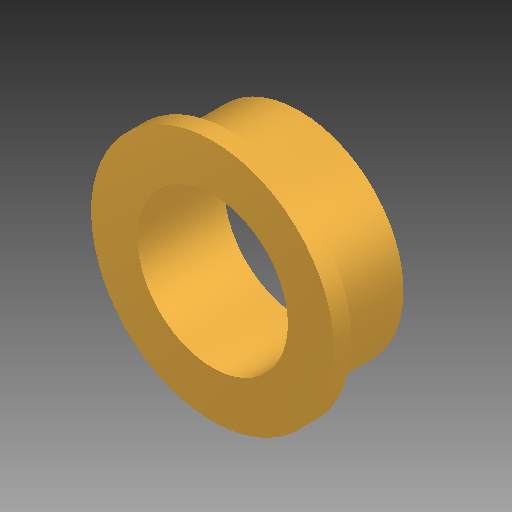
# Autodesk Inventor part: Thunderhex Bushing WCP-7348
Saved by Autodesk Inventor 2023 (Build 270158000, 158)
## iProperties
Created: 2022-01-15
Part Number: Thunderhex Bushing WCP-7348
Material: Bronze, Cast
Document SubType Name: Modeling
Density: 8.87 g/cm^3
Appearance: Brass - Satin
Mass: 11.062 g
Surface Area: 13.1267 cm^2
Volume: 1.24713 cm^3
Autodesk Inventor part; units mm, degrees
ref_plane "YZ Plane" through (0, 0, 0) normal (1, 0, 0) x (0, 1, 0)
ref_plane "XZ Plane" through (0, 0, 0) normal (0, 1, 0) x (-1, 0, 0)
ref_plane "XY Plane" through (0, 0, 0) normal (0, 0, 1) x (1, 0, 0)
sketch "Sketch1" plane through (0, 0, 0) normal (1, 0, 0) x (0, 1, 0)
  line L0 (0, 0) -> (9.525, 0)
  line L1 (9.525, 0) -> (9.525, 6.35)
  line L2 (9.525, 6.35) -> (11.1125, 6.35)
  line L3 (11.1125, 6.35) -> (11.1125, 7.9375)
  line L4 (11.1125, 7.9375) -> (0, 7.9375)
  line L5 (0, 7.9375) -> (0, 0) construction
  line L6 (6.875, 7.9375) -> (6.875, 0)
  dimension "d0" = 22.225
  dimension "d1" = 19.05
  dimension "d2" = 13.75
  dimension "d3" = 7.9375
  dimension "d4" = 6.35
  constraints: 14 end point, 6 perpendicular, 2 point on line, 1 horizontal
  measures "d0" diameter of L3 L5
  measures "d1" diameter of L1 L5
  measures "d2" diameter of L6 L5
  measures "d3" distance between parallel lines of L4 L0
  measures "d4" distance of L0.end L1.end
revolve "Revolution1" add sketch "Sketch1" angle 360 about axis through (0, 0, 7.9375) along (0, 0, -1)
body "Solid1"
